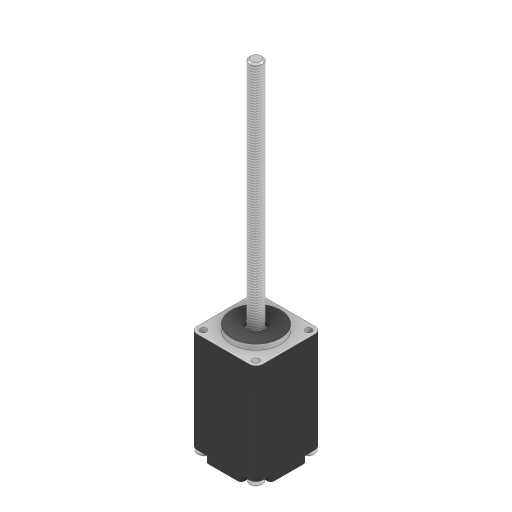
# Autodesk Inventor part: Nema 8
Saved by Autodesk Inventor 2023 (Build 270158000, 158)
## iProperties
Created: 2022-03-01
Part Number: Nema 8
Material: Generic
Document SubType Name: Modeling
Designer: ferrerx
Density: 1 g/cm^3
Appearance: Default
Author: ferrerx
Autodesk Inventor part; units mm, degrees
ref_plane "YZ Plane" through (0, 0, 0) normal (1, 0, 0) x (0, 1, 0)
ref_plane "XZ Plane" through (0, 0, 0) normal (0, 1, 0) x (-1, 0, 0)
ref_plane "XY Plane" through (0, 0, 0) normal (0, 0, 1) x (1, 0, 0)
sketch "Sketch1" plane through (0, 0, 0) normal (0, 1, 0) x (-1, 0, 0)
  line L0 (10, 10) -> (-10, 10)
  line L1 (-10, 10) -> (-10, -10)
  line L2 (-10, -10) -> (10, -10)
  line L3 (10, -10) -> (10, 10)
  line L4 (10, 10) -> (-10, -10) construction
  line L5 (-10, 10) -> (10, -10) construction
  point P0 (0, 0)
  dimension "d0" = 20
  dimension "d1" = 20
  constraints: 12 end point, 2 midpoint, 2 parallel, 1 horizontal, 1 perpendicular
  measures "d0" distance of L1.end L2.end
  measures "d1" distance of L0.end L1.end
extrude "Extrusion1" add sketch "Sketch1" along normal blind 32.5
sketch "Sketch2" plane through (0, 32.5, 0) normal (0, 1, 0) x (1, 0, 0)
  circle A0 centre (0, 0) radius 7.5
  dimension "d4" = 15
  constraints: 1 centre point, 1 coincident
  measures "d4" diameter of A0
extrude "Extrusion2" add sketch "Sketch2" along normal blind 1.6
sketch "Sketch3" plane through (0, 34.1, 0) normal (0, 1, 0) x (1, 0, 0)
  circle A0 centre (0, 0) radius 2
  dimension "d7" = 4
  constraints: 1 centre point, 1 coincident
  measures "d7" diameter of A0
extrude "Extrusion3" add sketch "Sketch3" along normal blind 70
sketch "Sketch5" plane through (0, 34.1, 0) normal (0, 1, 0) x (1, 0, 0)
  circle A0 centre (0, 0) radius 2 projected
  circle A1 centre (0, 0) radius 2.75
  dimension "d10" = 5.5
  constraints: 1 centre point, 1 coincident
  measures "d10" diameter of A1
extrude "Extrusion4" cut sketch "Sketch5" against normal blind 1.6
chamfer "Chamfer1" distance 0.5 angle 45 1 edges at (-2, 104.1, 0)
sketch "Sketch6" plane through (0, 32.5, 0) normal (0, 1, 0) x (1, 0, 0)
  line L0 (-8, -8) -> (8, -8) construction
  line L1 (8, -8) -> (8, 8) construction
  line L2 (8, 8) -> (-8, 8) construction
  line L3 (-8, 8) -> (-8, -8) construction
  line L4 (-8, -8) -> (8, 8) construction
  line L5 (8, -8) -> (-8, 8) construction
  circle A0 centre (-8, 8) radius 1
  circle A1 centre (8, 8) radius 1
  circle A2 centre (8, -8) radius 1
  circle A3 centre (-8, -8) radius 1
  point P0 (0, 0)
  dimension "d16" = 16
  dimension "d17" = 16
  dimension "d18" = 2
  dimension "d19" = 2
  dimension "d20" = 2
  dimension "d21" = 2
  constraints: 12 end point, 4 centre point, 4 coincident, 2 midpoint, 2 parallel, 1 horizontal, 1 perpendicular
  measures "d16" distance of L0.end L1.end
  measures "d17" distance of L1.end L2.end
  measures "d18" diameter of A0
  measures "d19" diameter of A1
  measures "d20" diameter of A2
  measures "d21" diameter of A3
extrude "Extrusion5" cut sketch "Sketch6" against normal blind 3
sketch "Sketch7" plane through (0, 0, 0) normal (0, -1, 0) x (1, 0, 0)
  circle A0 centre (0, 0) radius 2.7
  dimension "d24" = 5.4
  constraints: 1 centre point, 1 coincident
  measures "d24" diameter of A0
extrude "Extrusion6" cut sketch "Sketch7" against normal blind 3
sketch "Sketch8" plane through (0, 0, 0) normal (0, -1, 0) x (1, 0, 0)
  line L0 (10, -10) -> (5.5, -10)
  line L1 (5.5, -10) -> (5.5, -5.5)
  line L2 (5.5, -5.5) -> (10, -5.5)
  line L3 (10, -5.5) -> (10, -10)
  line L4 (-10, -10) -> (-5.5, -10)
  line L5 (-5.5, -10) -> (-5.5, -5.5)
  line L6 (-5.5, -5.5) -> (-10, -5.5)
  line L7 (-10, -5.5) -> (-10, -10)
  line L8 (10, 10) -> (10, -10) projected
  line L9 (10, 10) -> (5.5, 10)
  line L10 (5.5, 10) -> (5.5, 5.5)
  line L11 (5.5, 5.5) -> (10, 5.5)
  line L12 (10, 5.5) -> (10, 10)
  line L13 (-10, 10) -> (10, 10) projected
  line L14 (-10, 10) -> (-5.5, 10)
  line L15 (-5.5, 10) -> (-5.5, 5.5)
  line L16 (-5.5, 5.5) -> (-10, 5.5)
  line L17 (-10, 5.5) -> (-10, 10)
  line L18 (10, -10) -> (-10, -10) projected
  point P0 (0, 0)
  dimension "d27" = 11
  dimension "d28" = 11
  dimension "d29" = 5.5
  dimension "d30" = 11
  dimension "d31" = 5.5
  dimension "d32" = 11
  constraints: 32 end point, 8 parallel, 4 horizontal, 4 perpendicular, 2 point on line, 1 collinear
  measures "d27" distance between parallel lines of L16 L6
  measures "d28" distance between parallel lines of L1 L5
  measures "d29" distance from line of point (0, 0) L1
  measures "d30" distance between parallel lines of L2 L11
  measures "d31" distance from line of point (0, 0) L2
  measures "d32" distance between parallel lines of L15 L10
extrude "Extrusion7" cut sketch "Sketch8" against normal blind 2
sketch "Sketch9" plane through (0, 2, 0) normal (0, -1, 0) x (1, 0, 0)
  circle A0 centre (8, -8) radius 1.9
  circle A1 centre (-8, -8) radius 1 projected
  circle A2 centre (-8, -8) radius 1.9
  circle A3 centre (-8, 8) radius 1 projected
  circle A4 centre (-8, 8) radius 1.9
  circle A5 centre (8, 8) radius 1 projected
  circle A6 centre (8, 8) radius 1.9
  point P0 (0, 0)
  dimension "d35" = 3.8
  dimension "d36" = 3.8
  dimension "d37" = 3.8
  dimension "d38" = 3.8
  constraints: 4 centre point, 3 coincident
  measures "d35" diameter of A0
  measures "d36" diameter of A2
  measures "d37" diameter of A4
  measures "d38" diameter of A6
extrude "Extrusion8" add sketch "Sketch9" along normal blind 1.6 contours A0 | A1 | A2 | A3 | A4 | A5 | A6
fillet "Fillet1" radius 0.5 4 edges at (-9.9, 0.4, -8) (6.1, 0.4, -8) (6.1, 0.4, 8) (-9.9, 0.4, 8)
fillet "Fillet2" radius 2 4 edges at (-10, 17.25, -10) (10, 17.25, -10) (-10, 17.25, 10) (10, 17.25, 10)
fillet "Fillet3" radius 1 12 edges at (5.5, 1, -10) (-5.5, 1, -5.5) (-5.5, 1, -10) (-10, 1, -5.5) (-10, 1, 5.5) (-5.5, 1, 10) (-5.5, 1, 5.5) (5.5, 1, 10) (5.5, 1, 5.5) (10, 1, 5.5) (5.5, 1, -5.5) (10, 1, -5.5)
thread "Thread1" size "M4x0.7" class "6g" standard "ANSI Metric M Profile" full length
body "Solid1"
